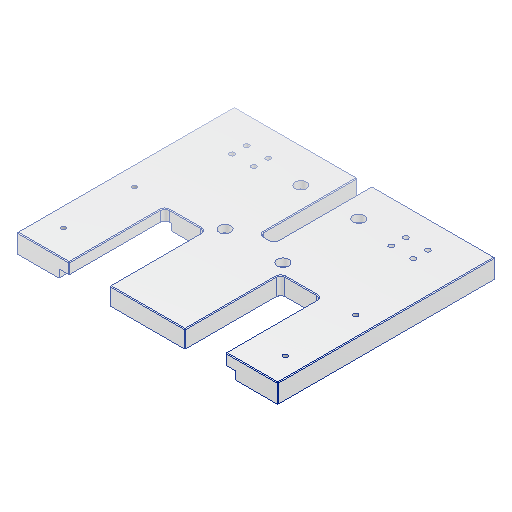
# Autodesk Inventor part: Chapa superior guia berço v1.2
Saved by Autodesk Inventor 2026.1 (Build 301233020, 233B)
## iProperties
Created: 2025-10-01
Part Number: Chapa superior guia berço v1.2
Material: Aluminio 1060
Document SubType Name: Modeling
Designer: Willian Pinheiro
Mass: 721.159 g
Surface Area: 628.173 cm^2
Volume: 267.096 cm^3
Density: 2.7 g/cm^3
Appearance: Alumínio - Plano
Description: Chapa superior guia berço v1.2
Dimensões: 13,5 x 150 x 180 mm
Total: 2
Author: Willian Pinheiro
Revision Number: 01
Autodesk Inventor part; units mm, degrees
ref_plane "YZ Plane" through (0, 0, 0) normal (1, 0, 0) x (0, 1, 0)
ref_plane "XZ Plane" through (0, 0, 0) normal (0, 1, 0) x (-1, 0, 0)
ref_plane "XY Plane" through (0, 0, 0) normal (0, 0, 1) x (1, 0, 0)
sketch "Esboço1" plane through (0, 0, 0) normal (0, 0, 1) x (1, 0, 0)
  line L0 (-126, 0) -> (126, 0) construction
  line L1 (0, -107.2) -> (0, 111.2) construction
  line L2 (-90, 75) -> (90, 75)
  line L3 (90, 75) -> (90, -75)
  line L4 (90, -75) -> (-90, -75)
  line L5 (-90, -75) -> (-90, 75)
  line L6 (-62.5, 56) -> (-47.5, 56) construction
  line L7 (-47.5, 56) -> (-47.5, 46) construction
  line L8 (-47.5, 46) -> (-62.5, 46) construction
  line L9 (-62.5, 46) -> (-62.5, 56) construction
  line L10 (-55, 56) -> (-55, 46) construction
  line L11 (-62.5, 51) -> (-47.5, 51) construction
  line L12 (-65, 65.5) -> (-45, 65.5) construction
  line L13 (-45, 65.5) -> (-45, 36.5) construction
  line L14 (-45, 36.5) -> (-65, 36.5) construction
  line L15 (-65, 36.5) -> (-65, 65.5) construction
  line L16 (-44, 66.5) -> (-66, 66.5)
  line L17 (-66, 66.5) -> (-66, 35.5)
  line L18 (-66, 35.5) -> (-44, 35.5)
  line L19 (-44, 35.5) -> (-44, 66.5)
  circle A0 centre (-66, 63.5) radius 3
  circle A1 centre (-44, 63.5) radius 3
  circle A2 centre (-66, 38.5) radius 3
  circle A3 centre (-44, 38.5) radius 3
  line L20 (-60, 75) -> (-50, 75) construction
  line L21 (-50, 75) -> (-50, -75) construction
  line L22 (-50, -75) -> (-60, -75) construction
  line L23 (-60, -75) -> (-60, 75) construction
  line L24 (-61, 76) -> (-49, 76)
  line L25 (-49, 76) -> (-49, -76)
  line L26 (-49, -76) -> (-61, -76)
  line L27 (-61, -76) -> (-61, 76)
  line L28 (62.5, 56) -> (47.5, 56) construction
  line L29 (47.5, 56) -> (47.5, 46) construction
  line L30 (47.5, 46) -> (62.5, 46) construction
  line L31 (62.5, 46) -> (62.5, 56) construction
  line L32 (55, 56) -> (55, 46) construction
  line L33 (62.5, 51) -> (47.5, 51) construction
  line L34 (65, 65.5) -> (45, 65.5) construction
  line L35 (45, 65.5) -> (45, 36.5) construction
  line L36 (45, 36.5) -> (65, 36.5) construction
  line L37 (65, 36.5) -> (65, 65.5) construction
  line L38 (44, 66.5) -> (66, 66.5)
  line L39 (66, 66.5) -> (66, 35.5)
  line L40 (66, 35.5) -> (44, 35.5)
  line L41 (44, 35.5) -> (44, 66.5)
  circle A4 centre (66, 63.5) radius 3
  circle A5 centre (44, 63.5) radius 3
  circle A6 centre (66, 38.5) radius 3
  circle A7 centre (44, 38.5) radius 3
  line L42 (60, 75) -> (50, 75) construction
  line L43 (50, 75) -> (50, -75) construction
  line L44 (50, -75) -> (60, -75) construction
  line L45 (60, -75) -> (60, 75) construction
  line L46 (61, 76) -> (49, 76)
  line L47 (49, 76) -> (49, -76)
  line L48 (49, -76) -> (61, -76)
  line L49 (61, -76) -> (61, 76)
  line L50 (-54, -9) -> (-26, -9)
  line L51 (-26, -9) -> (-26, -75)
  line L52 (-26, -75) -> (-54, -75)
  line L53 (-54, -75) -> (-54, -9)
  line L54 (-40, -9) -> (-40, -75) construction
  line L55 (54, -9) -> (26, -9)
  line L56 (26, -9) -> (26, -75)
  line L57 (26, -75) -> (54, -75)
  line L58 (54, -75) -> (54, -9)
  line L59 (40, -9) -> (40, -75) construction
  line L60 (0, 75) -> (0, 12.5) construction
  line L61 (5, 75) -> (5, 12.5)
  line L62 (-5, 12.5) -> (-5, 75)
  arc A8 (5, 75) -> (-5, 75) centre (0, 75) ccw
  arc A9 (-5, 12.5) -> (5, 12.5) centre (0, 12.5) ccw
  line L63 (-20, 51) -> (20, 51) construction
  line L64 (20, 51) -> (20, -1.4) construction
  line L65 (20, -1.4) -> (-20, -1.4) construction
  line L66 (-20, -1.4) -> (-20, 51) construction
  line L67 (-20, 24.8) -> (20, 24.8) construction
  line L68 (-76.5, -7.5) -> (76.5, -7.5) construction
  line L69 (76.5, -7.5) -> (76.5, -56.4) construction
  line L70 (76.5, -56.4) -> (-76.5, -56.4) construction
  line L71 (-76.5, -56.4) -> (-76.5, -7.5) construction
  line L72 (-76.5, -31.95) -> (76.5, -31.95) construction
  line L73 (-25, 59) -> (-15, 59)
  line L74 (-15, 59) -> (-15, -9.4)
  line L75 (-15, -9.4) -> (-25, -9.4)
  line L76 (-25, -9.4) -> (-25, 59)
  line L77 (25, 59) -> (15, 59)
  line L78 (15, 59) -> (15, -9.4)
  line L79 (15, -9.4) -> (25, -9.4)
  line L80 (25, -9.4) -> (25, 59)
  line L81 (-5, 12.5) -> (5, 12.5)
  line L82 (5, 12.5) -> (5, 7.5)
  line L83 (5, 7.5) -> (-5, 7.5)
  line L84 (-5, 7.5) -> (-5, 12.5)
  point P0 (0, 0)
  point P1 (0, 43.75)
  point P2 (66, 41.5)
  point P3 (66, 60.5)
  point P4 (44, 60.5)
  point P5 (44, 41.5)
  point P6 (-66, 41.5)
  point P7 (-44, 41.5)
  point P8 (-44, 60.5)
  point P9 (-66, 60.5)
  point P10 (49, 75)
  point P11 (-49, 75)
  point P12 (-49, -75)
  point P13 (49, -9)
  point P14 (0, 7.5)
  dimension "d18" = 6
  dimension "d0" = 180
  dimension "d1" = 150
  dimension "d2" = 10
  dimension "d3" = 15
  dimension "d4" = 20
  dimension "d5" = 29
  dimension "d6" = 10
  dimension "d7" = 1
  dimension "d8" = 110
  dimension "d9" = 80
  dimension "d10" = 28
  dimension "d11" = 66
  dimension "d12" = 10
  dimension "d13" = 62.5
  dimension "d14" = 52.4
  dimension "d15" = 40
  dimension "d16" = 24
  dimension "d17" = 1
  dimension "d19" = 153
  dimension "d20" = 48.9
  dimension "d21" = 18.6
  dimension "d26" = 68.4
  dimension "d27" = 10
  constraints: 168 end point, 41 symmetric about line, 23 parallel, 12 midpoint, 11 perpendicular, 9 horizontal, 8 centre point, 5 tangent, 4 point on circle, 4 point on line, 3 collinear, 1 vertical, 28 other
  measures "d0" distance between parallel lines of L3 L5
  measures "d1" distance between parallel lines of L4 L2
  measures "d2" distance of L8.end L6.start
  measures "d3" distance of L6.start L6.end
  measures "d4" distance of L13.end L14.end
  measures "d5" distance of L14.end L12.start
  measures "d6" distance between parallel lines of L21 L23
  measures "d7" distance between parallel lines of L27 L23
  measures "d8" distance between parallel lines of L32 L10
  measures "d9" distance between parallel lines of L59 L54
  measures "d10" distance between parallel lines of L51 L53
  measures "d11" distance of L50.end L51.end
  measures "d12" distance between parallel lines of L61 L62
  measures "d13" distance from line of L2 L60.end
  measures "d14" distance of L65.end L63.start
  measures "d15" distance of L64.end L65.end
  measures "d16" distance between parallel lines of L63 L2
  measures "d17" distance between parallel lines of L16 L12
  measures "d19" distance between parallel lines of L69 L71
  measures "d20" distance between parallel lines of L68 L70
  measures "d21" distance between parallel lines of L4 L70
  measures "d26" distance between parallel lines of L75 L73
  measures "d27" distance between parallel lines of L74 L76
extrude "Extrusão1" add sketch "Esboço1" against normal blind 13.5 contours L62 L84 L83 L82 L61 L2 L47 L38 A5 L41 A7 L40 L55 L56 L4 L51 L50 L25 L18 A3 L19 A1 L16 | L2 L61 L81 L62 | L25 L16 L27 L2 | L81 A9 | A9 L83 L84 | L2 L49 L38 L47 | L82 L83 A9 | L27 L16 A0 L17 A2 L18 L4 L5 L2 | L25 L18 L27 L16 | L16 A1 L19 A3 L18 L25 | L2 L3 L4 L49 L40 A6 L39 A4 L38 | L47 L40 A7 L41 A5 L38 | L38 L49 L40 L47 | L27 L18 A2 L17 A0 L16 | A1 L19 | L19 A1 | L25 L50 L53 L4 L27 L18 | L38 A4 L39 A6 L40 L49 | A5 L41 | L41 A5 | L40 L49 L4 L58 L55 L47 | A0 L17 | L17 A0 | A3 L19 | L19 A3 | L50 L51 L4 L25 | L25 L4 L53 L50 | A4 L39 | L39 A4 | A7 L41 | L41 A7 | L55 L58 L4 L47 | L47 L4 L56 L55 | A2 L17 | L17 A2 | A6 L39 | L39 A6 | L73 L74 L75 L76 | L80 L79 L78 L77
extrude "Extrusão2" cut sketch "Esboço1" against normal through all contours A8 L2 | L2 L61 L81 L62 | L81 A9 | A9 L83 L84 | L82 L83 A9 | L50 L51 L4 L25 | L25 L4 L53 L50 | L55 L58 L4 L47 | L47 L4 L56 L55
extrude "Extrusão3" cut sketch "Esboço1" along normal blind 1 from surface at -13.5 contours L62 L84 L83 L82 L61 L2 L47 L38 A5 L41 A7 L40 L55 L56 L4 L51 L50 L25 L18 A3 L19 A1 L16 | L2 L61 L81 L62 | L81 A9 | A9 L83 L84 | L82 L83 A9 | L16 A1 L19 A3 L18 L25 | L47 L40 A7 L41 A5 L38 | A1 L19 | L19 A1 | A5 L41 | L41 A5 | A3 L19 | L19 A3 | L50 L51 L4 L25 | A7 L41 | L41 A7 | L55 L58 L4 L47 | L47 L4 L56 L55
extrude "Extrusão4" cut sketch "Esboço1" along normal blind 6 from surface at -13.5 contours L25 L16 L27 L2 | L2 L27 L24 L25 | L47 L46 L49 L2 | L2 L49 L38 L47 | L25 L18 L27 L16 | L38 L49 L40 L47 | L25 L50 L53 L4 L27 L18 | L40 L49 L4 L58 L55 L47 | L25 L4 L53 L50 | L55 L58 L4 L47 | L4 L25 L26 L27 | L49 L48 L47 L4
extrude "Extrusão5" cut sketch "Esboço1" along normal blind 9 from surface at -13.5 contours L25 L18 L27 L16 | L16 A1 L19 A3 L18 L25 | L47 L40 A7 L41 A5 L38 | L38 L49 L40 L47 | L27 L18 A2 L17 A0 L16 | A1 L19 | L19 A1 | L38 A4 L39 A6 L40 L49 | A5 L41 | L41 A5 | A0 L17 | L17 A0 | A3 L19 | L19 A3 | A4 L39 | L39 A4 | A7 L41 | L41 A7 | A2 L17 | L17 A2 | A6 L39 | L39 A6
hole "Furo1" at (-62.5, 56, 0) at (-62.5, 46, 0) at (-47.5, 46, 0) at (-47.5, 56, 0) at (47.5, 56, 0) at (47.5, 46, 0) at (62.5, 46, 0) at (62.5, 56, 0) direction (0, 0, -1) diameter 3.5 end through all clearance for "Countersunk Flat Head Hex Socket Screw ISO 10642" size "M3" standard "ISO"
hole "Furo2" at (-20, -1.4, 0) at (20, -1.4, 0) at (20, 51, 0) at (-20, 51, 0) direction (0, 0, -1) diameter 5 end through all counterbore diameter 8 counterbore depth 5 clearance for "Socket Head Cap Screw ISO 4762" size "M4" standard "ISO"
hole "Furo3" at (-76.5, -7.5, 0) at (76.5, -56.4, 0) at (76.5, -7.5, 0) at (-76.5, -56.4, 0) direction (0, 0, -1) diameter 3.242 end through all thread size "M4x0.7" class "6H" standard "ISO Metric profile"
fillet "Arredondamento1" radius 3 6 edges at (-54, -9, -3.75) (-26, -9, -6.25) (26, -9, -6.25) (54, -9, -3.75) (-5, 7.5, -6.25) (5, 7.5, -6.25)
fillet "Arredondamento1" radius 1 16 edges at (66, 60.5, -9) (66, 41.5, -9) (44, 41.5, -8.5) (44, 60.5, -8.5) (-44, 60.5, -8.5) (-66, 60.5, -9) (-66, 41.5, -9) (-44, 41.5, -8.5) (25, -9.4, -13) (15, -9.4, -13) (15, 59, -13) (25, 59, -13) (-15, -9.4, -13) (-15, 59, -13) (-25, 59, -13) (-25, -9.4, -13)
chamfer "Chanfro1" distance 0.5 angle 45 88 edges at (90, 0, 0) (90, 75, -6.75) (-47.5, 75, 0) (47.5, 75, 0) (27, 75, -12.5) (-27, 75, -12.5) (-90, 75, -6.75) (-90, 0, 0) (-90, -75, -6.75) (-72, -75, 0) (0, -75, -12.5) (0, -75, 0) (72, -75, 0) (-54, -75, -3.75) (54, -75, -3.75) (-54, -43.5, 0) (-53.1213, -9.8787, 0) (-40, -9, 0) (-26.8787, -9.8787, 0) (-26, -43.5, 0) (26, -43.5, 0) (26.8787, -9.8787, 0) (40, -9, 0) (53.1213, -9.8787, 0) (54, -43.5, 0) (-46.5, 35.5, -12.5) (-41.0239, 38.122, -12.5) (-43.7906, 41.7606, -12.5) (-44, 51, -12.5) (-43.7906, 60.2394, -12.5) (-41.0239, 63.878, -12.5) (-46.5, 66.5, -12.5) (-49, 13.25, -12.5) (-39, -9, -12.5) (-26.8787, -9.8787, -12.5) (-26, -43.5, -12.5) (26, -43.5, -12.5) (26.8787, -9.8787, -12.5) (39, -9, -12.5) (46.5, 35.5, -12.5) (41.0239, 38.122, -12.5) (43.7906, 41.7606, -12.5) (44, 51, -12.5) (43.7906, 60.2394, -12.5) (41.0239, 63.878, -12.5) (46.5, 66.5, -12.5) (49, 13.25, -12.5) (49, 70.75, -12.5) (-49, 70.75, -12.5) (-75.5, -75, -13.5) (-61, -19.75, -13.5) (-63.5, 35.5, -13.5) (-68.9761, 38.122, -13.5) (-66.2094, 41.7606, -13.5) (-66, 51, -13.5) (-66.2094, 60.2394, -13.5) (-68.9761, 63.878, -13.5) (-63.5, 66.5, -13.5) (-61, 70.75, -13.5) (61, -19.75, -13.5) (75.5, -75, -13.5) (90, -75, -6.75) (90, 0, -13.5) (75.5, 75, -13.5) (68.9761, 38.122, -13.5) (66.2094, 41.7606, -13.5) (66, 51, -13.5) (66.2094, 60.2394, -13.5) (68.9761, 63.878, -13.5) (63.5, 66.5, -13.5) (63.5, 35.5, -13.5) (-5, 42.75, 0) (-4.1213, 8.3787, 0) (0, 7.5, 0) (4.1213, 8.3787, 0) (5, 42.75, 0) (-5, 42.75, -12.5) (-4.1213, 8.3787, -12.5) (0, 7.5, -12.5) (4.1213, 8.3787, -12.5) (5, 42.75, -12.5) (-5, 75, -6.25) (5, 75, -6.25) (61, 70.75, -13.5) (-26, -75, -6.25) (26, -75, -6.25) (-75.5, 75, -13.5) (-90, 0, -13.5)
